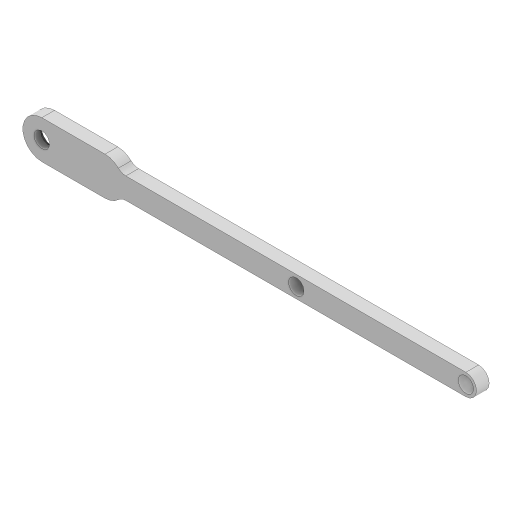
# Autodesk Inventor part: 200_forservo
Saved by Autodesk Inventor 2023 (Build 270158000, 158)
## iProperties
Created: 2023-04-16
Part Number: 200_forservo
Material: 一般
Document SubType Name: Modeling
Designer: JOU
Density: 1 g/cm^3
Appearance: 預設
Author: JOU
Autodesk Inventor part; units mm, degrees
ref_plane "YZ Plane" through (0, 0, 0) normal (1, 0, 0) x (0, 1, 0)
ref_plane "XZ Plane" through (0, 0, 0) normal (0, 1, 0) x (-1, 0, 0)
ref_plane "XY Plane" through (0, 0, 0) normal (0, 0, 1) x (1, 0, 0)
sketch "草圖1" plane through (0, 0, 0) normal (0, 0, 1) x (1, 0, 0)
  line L0 (-200, 0) -> (0, 0) construction
  line L1 (-200, -5) -> (0, -5)
  line L2 (0, 5) -> (-200, 5)
  arc A0 (-200, 5) -> (-200, -5) centre (-200, 0) ccw
  arc A1 (0, -5) -> (0, 5) centre (0, 0) ccw
  circle A2 centre (0, 0) radius 3.65
  circle A3 centre (-80, 0) radius 3.65
  circle A4 centre (-200, 0) radius 3.65
  point P0 (-100, 0)
  dimension "d0" = 200
  dimension "d1" = 10
  dimension "d3" = 7.3
  dimension "d27" = 7.3
  dimension "d47" = 7.3
  constraints: 8 end point, 5 centre point, 4 point on circle, 4 tangent, 3 coincident, 1 horizontal, 1 midpoint, 1 parallel, 1 point on line
  measures "d0" distance of L2.start L2.end
  measures "d1" distance between parallel lines of L1 L2
  measures "d3" diameter of A2
  measures "d27" diameter of A3
  measures "d47" diameter of A4
extrude "擠出1" add sketch "草圖1" along normal blind 6 contours A0 L2 A1 L1 | A4
sketch "草圖4" plane through (0, 0, 0) normal (0, 0, -1) x (-1, 0, 0)
  line L0 (200, 0) -> (170.2, 0) construction
  line L1 (200, -9) -> (170.2, -9)
  line L2 (170.2, 9) -> (200, 9)
  arc A0 (200, -9) -> (200, 9) centre (200, 0) ccw
  arc A1 (170.2, 9) -> (170.2, -9) centre (170.2, 0) ccw
  arc A2 (200, -5) -> (200, 5) centre (200, 0) ccw projected
  circle A3 centre (170.2, 0) radius 0.6
  circle A4 centre (170.2, 0) radius 4.4
  circle A5 centre (200, 0) radius 6.65
  line L3 (169.8678, 4.3874) -> (199.4979, 6.631)
  line L4 (169.8678, -4.3874) -> (199.4979, -6.631)
  point P0 (0, 0)
  point P1 (185.1, 0)
  dimension "d31" = 9
  dimension "d36" = 1.2
  dimension "d37" = 29.8
  dimension "d42" = 8.8
  dimension "d44" = 13.3
  constraints: 12 end point, 8 point on circle, 7 tangent, 5 centre point, 4 coincident, 1 concentric, 1 horizontal alignment, 1 midpoint, 1 parallel, 1 other
  measures "d31" radius of A0
  measures "d36" diameter of A3
  measures "d37" distance of A3.centre L0.start
  measures "d42" diameter of A4
  measures "d44" diameter of A5
extrude "擠出5" add sketch "草圖4" against normal blind 6 contours L1 A1 L2 A0 | A3 | A4 | A4 L3 A5 L4 | A5
extrude "擠出6" cut sketch "草圖4" against normal blind 2.9 contours A3 | A4 | A4 L3 A5 L4 | A5
extrude "擠出7" cut sketch "草圖1" along normal through all contours A4
fillet "圓角1" radius 5 2 edges at (-162.7167, 5, 3) (-162.7167, -5, 3)
